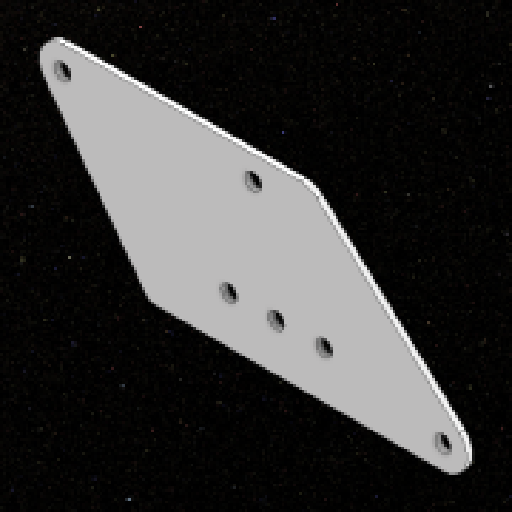
# Autodesk Inventor part: sled
Saved by Autodesk Inventor 2024 (Build 280153000, 153)
## iProperties
Created: 2024-02-24
Part Number: sled
Material: Acetal Resin, White
Document SubType Name: Modeling
Designer: Averey Ku
Density: 1.425 g/cm^3
Appearance: Smooth - White
Author: Averey Ku
Autodesk Inventor part; units mm, degrees
ref_plane "YZ Plane" through (0, 0, 0) normal (1, 0, 0) x (0, 1, 0)
ref_plane "XZ Plane" through (0, 0, 0) normal (0, 1, 0) x (-1, 0, 0)
ref_plane "XY Plane" through (0, 0, 0) normal (0, 0, 1) x (1, 0, 0)
sketch "main" plane through (0, 0, 0) normal (0, 0, 1) x (1, 0, 0)
  circle A0 centre (-89.308, 4.2536) radius 2.1844
  circle A1 centre (-53.9639, 105.8536) radius 2.1844
  line L0 (-48.895, 26.3761) -> (-85.5202, -0.8431)
  line L1 (-47.6139, 28.9244) -> (-47.6139, 105.8536)
  arc A2 (-47.6139, 105.8536) -> (-58.6192, 110.1722) centre (-53.9639, 105.8536) ccw
  line L2 (-58.6192, 110.1722) -> (-93.9633, 72.0722)
  arc A3 (-48.895, 26.3761) -> (-47.6139, 28.9244) centre (-50.7889, 28.9244) ccw
  arc A4 (-95.658, 4.2536) -> (-85.5202, -0.8431) centre (-89.308, 4.2536) ccw
  arc A5 (-93.9633, 72.0722) -> (-95.658, 67.7536) centre (-89.308, 67.7536) ccw
  line L3 (-95.658, 67.7536) -> (-95.658, 4.2536)
  circle A6 centre (-89.308, 55.0536) radius 2.1844
  point P0 (1.1183, 5.4838)
  dimension "d8" = 3.175
  dimension "d11" = 4.3688
  measures "d8" radius of A3
  measures "d11" diameter of A6
sketch "Sketch1" plane through (0, 0, 0) normal (0, 0, 1) x (1, 0, 0)
  circle A0 centre (-44.45, 6.35) radius 2.0955
  circle A1 centre (-57.15, 6.35) radius 2.0955
  circle A2 centre (-31.75, 6.35) radius 2.0955
  circle A3 centre (-101.6, 35.3441) radius 2.1844
  circle A4 centre (0, 0) radius 2.1844
  line L0 (-79.4775, -5.0689) -> (-106.6966, 31.5564)
  line L1 (-76.9292, -6.35) -> (0, -6.35)
  arc A5 (0, -6.35) -> (4.3186, 4.6553) centre (0, 0) ccw
  line L2 (4.3186, 4.6553) -> (-33.7814, 39.9994)
  arc A6 (-79.4775, -5.0689) -> (-76.9292, -6.35) centre (-76.9292, -3.175) ccw
  arc A7 (-101.6, 41.6941) -> (-106.6966, 31.5564) centre (-101.6, 35.3441) ccw
  arc A8 (-33.7814, 39.9994) -> (-38.1, 41.6941) centre (-38.1, 35.3441) ccw
  line L3 (-38.1, 41.6941) -> (-101.6, 41.6941)
  circle A9 centre (-50.8, 35.3441) radius 2.1844
  dimension "d12" = 4.191
  dimension "d13" = 4.191
  dimension "d14" = 4.191
  constraints: 3 centre point, 1 other
  measures "d12" diameter of A0
  measures "d13" diameter of A1
  measures "d14" diameter of A2
extrude "Extrusion1" add sketch "Sketch1" along normal blind 1.5875
body "Solid1"
